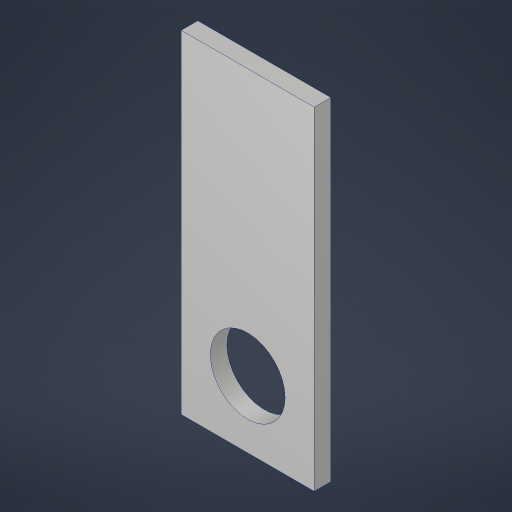
# Autodesk Inventor part: CL6-003
Saved by Autodesk Inventor 2023.4 (Build 274418000, 418)
## iProperties
RuleStatus: InUse
Created: 2025-03-15
Part Number: CL6-003
Material: Aluminum 6061
Document SubType Name: Modeling
Designer: brand
Mass: 132.735 g
Surface Area: 177.419 cm^2
Volume: 49.1612 cm^3
Density: 2.7 g/cm^3
Appearance: Aluminum - Flat
AfterDocNew0: SHOW
AfterDocOpen0: SHOW
Author: brand
Autodesk Inventor part; units mm, degrees
ref_plane "YZ Plane" through (0, 0, 0) normal (1, 0, 0) x (0, 1, 0)
ref_plane "XZ Plane" through (0, 0, 0) normal (0, 1, 0) x (-1, 0, 0)
ref_plane "XY Plane" through (0, 0, 0) normal (0, 0, 1) x (1, 0, 0)
sketch "Sketch1" plane through (0, 0, 0) normal (0, 0, 1) x (1, 0, 0)
  line L0 (-25.4, -63.5) -> (25.4, -63.5)
  line L1 (25.4, -63.5) -> (25.4, 63.5)
  line L2 (25.4, 63.5) -> (-25.4, 63.5)
  line L3 (-25.4, 63.5) -> (-25.4, -63.5)
  line L4 (-25.4, -63.5) -> (25.4, 63.5) construction
  line L5 (25.4, -63.5) -> (-25.4, 63.5) construction
  point P0 (0, 0)
  dimension "width" = 50.8
  dimension "length" = 127
  constraints: 12 end point, 2 midpoint, 2 parallel, 1 horizontal, 1 perpendicular
  measures "width" distance of L2.end L1.end
  measures "length" distance of L0.end L1.end
extrude "Extrusion1" add sketch "Sketch1" along normal mid plane 6.35
sketch "Sketch2" plane through (0, 0, 3.175) normal (0, 0, 1) x (1, 0, 0)
  line L0 (-25.4, -63.5) -> (-25.4, 63.5) construction
  line L1 (-25.4, 63.5) -> (25.4, 63.5) construction
  line L2 (25.4, 63.5) -> (25.4, -63.5) construction
  line L3 (25.4, -63.5) -> (-25.4, -63.5) construction
  point P0 (0, 0)
  point P1 (0, -38.1)
  point P2 (0, -63.5)
  dimension "d4" = 25.4
  constraints: 1 midpoint, 1 vertical alignment
  measures "d4" distance from line of L3 point (0, -38.1)
hole "Hole1" at (0, -38.1, 3.175) direction (0, 0, -1) diameter 28.575 end through all
body "Solid1"
